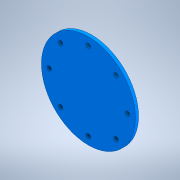
# Autodesk Inventor part: B-01
Saved by Autodesk Inventor 2021 (Build 250183000, 183)
## iProperties
Created: 2022-03-08
Part Number: B-01
Material: PETG
Document SubType Name: Modeling
Designer: Alcatraz
Density: 1.27 g/cm^3
Appearance: Genérico
Author: Alcatraz
Autodesk Inventor part; units mm, degrees
ref_plane "YZ Plane" through (0, 0, 0) normal (1, 0, 0) x (0, 1, 0)
ref_plane "XZ Plane" through (0, 0, 0) normal (0, 1, 0) x (-1, 0, 0)
ref_plane "XY Plane" through (0, 0, 0) normal (0, 0, 1) x (1, 0, 0)
sketch "Boceto1" plane through (0, 0, 0) normal (0, 0, 1) x (1, 0, 0)
  circle A0 centre (-35.3566, -35.354) radius 2.75
  circle A1 centre (-35.3547, 35.356) radius 2.75
  circle A2 centre (-50, 0) radius 2.75
  circle A3 centre (0, 50) radius 2.75
  circle A4 centre (0, -50) radius 2.75
  circle A5 centre (35.356, 35.3547) radius 2.75
  circle A6 centre (35.3561, -35.3546) radius 2.75
  circle A7 centre (0, 0) radius 45
  circle A8 centre (0, 0) radius 60
  circle A9 centre (50, 0) radius 2.75
  dimension "d0" = 120
  dimension "d1" = 5.5
  dimension "d2" = 5.5
  dimension "d3" = 5.5
  dimension "d4" = 5.5
  dimension "d5" = 5.5
  dimension "d6" = 5.5
  dimension "d7" = 5.5
  dimension "d8" = 5.5
  dimension "d9" = 50
  dimension "d10" = 7.25
  dimension "d11" = 50
  dimension "d12" = 50
  dimension "d13" = 50
  dimension "d14" = 50
  dimension "d15" = 50
  dimension "d16" = 50
  dimension "d17" = 50
  dimension "d21" = 90
  constraints: 10 centre point, 1 coincident
  measures "d0" diameter of A8
  measures "d1" diameter of A2
  measures "d2" diameter of A0
  measures "d3" diameter of A4
  measures "d4" diameter of A6
  measures "d5" diameter of A9
  measures "d6" diameter of A5
  measures "d7" diameter of A3
  measures "d8" diameter of A1
  measures "d9" distance of A5.centre point (0, 0)
  measures "d11" distance of point (0, 0) A3.centre
  measures "d12" distance of point (0, 0) A1.centre
  measures "d13" distance of A2.centre point (0, 0)
  measures "d14" distance of A0.centre point (0, 0)
  measures "d15" distance of point (0, 0) A4.centre
  measures "d16" distance of point (0, 0) A6.centre
  measures "d17" distance of point (0, 0) A9.centre
  measures "d21" diameter of A7
extrude "Extrusión1" add sketch "Boceto1" along normal blind 4 contours A7 | A8
equation "\"d1\" = DiametroTornillo"
equation "\"d2\" = DiametroTornillo"
equation "\"d3\" = DiametroTornillo"
equation "\"d4\" = DiametroTornillo"
equation "\"d5\" = DiametroTornillo"
equation "\"d6\" = DiametroTornillo"
equation "\"d7\" = DiametroTornillo"
equation "\"d8\" = DiametroTornillo"
equation "\"d11\" = d9"
equation "\"d12\" = d9"
equation "\"d13\" = d9"
equation "\"d14\" = d9"
equation "\"d15\" = d9"
equation "\"d16\" = d9"
equation "\"d17\" = d9"
equation "\"DiametroTornillo\" = 5.5"
